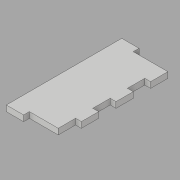
# Autodesk Inventor part: b_base_support 3
Saved by Autodesk Inventor 2019 (Build 230136000, 136)
## iProperties
Created: 2021-11-07
Part Number: b_base_support 3
Material: Generic
Document SubType Name: Modeling
Designer: Mohamed
Density: 1 g/cm^3
Appearance: Default
Author: Mohamed
Autodesk Inventor part; units mm, degrees
ref_plane "YZ Plane" through (0, 0, 0) normal (1, 0, 0) x (0, 1, 0)
ref_plane "XZ Plane" through (0, 0, 0) normal (0, 1, 0) x (-1, 0, 0)
ref_plane "XY Plane" through (0, 0, 0) normal (0, 0, 1) x (1, 0, 0)
sketch "Sketch1" plane through (0, 0, 0) normal (0, 1, 0) x (-1, 0, 0)
  line L0 (0, 0) -> (60, 0)
  line L1 (60, 0) -> (60, -133.4)
  line L2 (60, -133.4) -> (0, -133.4)
  line L3 (0, -133.4) -> (0, 0)
  dimension "d0" = 133.4
  dimension "d1" = 60
  constraints: 8 end point, 2 parallel, 1 horizontal, 1 perpendicular
  measures "d0" distance of L0.end L1.end
  measures "d1" distance of L0.start L0.end
extrude "Extrusion1" add sketch "Sketch1" along normal blind 6.7
sketch "Sketch2" plane through (0, 6.7, 0) normal (0, 1, 0) x (1, 0, 0)
  line L0 (0, 0) -> (0, 6.7)
  line L1 (0, 0) -> (0, 133.4) projected
  line L2 (0, 6.7) -> (-6.7, 6.7)
  line L3 (-6.7, 6.7) -> (-6.7, 26.7)
  line L4 (-6.7, 26.7) -> (0, 26.7)
  line L5 (0, 26.7) -> (0, 6.7)
  dimension "d4" = 6.7
  dimension "d5" = 6.7
  dimension "d6" = 20
  constraints: 10 end point, 2 parallel, 1 horizontal, 1 perpendicular, 1 point on line
  measures "d4" distance of L0.start L0.end
  measures "d5" distance of L3.end L4.end
  measures "d6" distance of L2.end L3.end
extrude "Extrusion2" cut sketch "Sketch2" against normal blind 6.7
pattern_linear "Rectangular Pattern1" count 3 spacing 40 along (0, 0, -1) of "Extrusion2"
sketch "Sketch3" plane through (0, 6.7, 0) normal (0, 1, 0) x (1, 0, 0)
  line L0 (0, 0) -> (-60, 0) projected
  line L1 (-60, 0) -> (-40, 0)
  line L2 (-40, 0) -> (-20, 0)
  line L3 (0, 6.7) -> (0, 0) projected
  line L4 (-40, 0) -> (0, 0)
  line L5 (0, 0) -> (0, 6.7)
  line L6 (0, 6.7) -> (-40, 6.7)
  line L7 (-40, 6.7) -> (-40, 0)
  line L8 (-60, 133.4) -> (-40, 133.4)
  line L9 (-60, 133.4) -> (0, 133.4) projected
  line L10 (0, 133.4) -> (0, 106.7) projected
  line L11 (-40, 133.4) -> (0, 133.4)
  line L12 (0, 133.4) -> (0, 126.7)
  line L13 (0, 126.7) -> (-40, 126.7)
  line L14 (-40, 126.7) -> (-40, 133.4)
  dimension "d12" = 20
  dimension "d15" = 20
  dimension "d16" = 6.7
  constraints: 22 end point, 4 parallel, 3 horizontal, 3 point on line, 2 perpendicular
  measures "d12" distance of L0.end L1.end
  measures "d15" distance of L8.start L8.end
  measures "d16" distance of L11.end L12.end
extrude "Extrusion3" cut sketch "Sketch3" against normal blind 6.7
body "Solid1"
